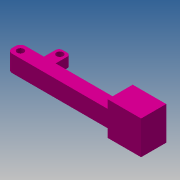
# Autodesk Inventor part: 連趕2
Saved by Autodesk Inventor 2015 (Build 190159000, 159)
## iProperties
Created: 2017-12-21
Part Number: 連趕2
Material: 一般
Document SubType Name: Modeling
Designer: user
Density: 1 g/cm^3
Appearance: 預設
Author: user
Autodesk Inventor part; units mm, degrees
ref_plane "YZ Plane" through (0, 0, 0) normal (1, 0, 0) x (0, 1, 0)
ref_plane "XZ Plane" through (0, 0, 0) normal (0, 1, 0) x (-1, 0, 0)
ref_plane "XY Plane" through (0, 0, 0) normal (0, 0, 1) x (1, 0, 0)
sketch "草圖1" plane through (0, 0, 0) normal (0, 0, 1) x (1, 0, 0)
  line L0 (0, 0) -> (80, 0)
  line L1 (80, 0) -> (80, 8)
  line L2 (60, 8) -> (0, 8)
  line L3 (0, 8) -> (0, 0)
  line L4 (80, 8) -> (60, 8)
  line L5 (60, 8) -> (60, 15)
  line L6 (60, 15) -> (80, 15)
  line L7 (80, 15) -> (80, 8)
  dimension "d0" = 80
  dimension "d1" = 20
  dimension "d2" = 15
  dimension "d3" = 8
  constraints: 16 end point, 4 parallel, 2 horizontal, 2 perpendicular
  measures "d0" distance of L0.start L0.end
  measures "d1" distance of L5.end L6.end
  measures "d2" distance between parallel lines of L0 L6
  measures "d3" distance between parallel lines of L0 L2
extrude "擠出1" add sketch "草圖1" along normal mid plane 20
sketch "草圖2" plane through (0, 0, 0) normal (0, 0, 1) x (1, 0, 0)
  line L0 (70, 31.4394) -> (70, 8.5)
  line L1 (60, 15) -> (80, 15) projected
  line L2 (80, 0) -> (80, 15) projected
  arc A0 (70, 8.5) -> (77.5, 16) centre (70, 16) ccw
  line L3 (70, 16) -> (77.5, 16)
  point P0 (0, 0)
  dimension "d14" = 7.5
  dimension "d15" = 1
  dimension "d16" = 10
  constraints: 6 end point, 2 point on circle, 1 centre point, 1 horizontal, 1 point on line, 1 vertical
  measures "d14" radius of A0
  measures "d15" distance between parallel lines of L1 L3
  measures "d16" distance between parallel lines of L2 L0
sketch "草圖3" plane through (0, 8, -10) normal (0, 1, 0) x (1, 0, 0)
  line L0 (60, 0) -> (60, -20) projected
  line L1 (0, 0) -> (60, 0)
  line L2 (60, 0) -> (60, -5)
  line L3 (60, -5) -> (0, -5)
  line L4 (0, -5) -> (0, 0)
  line L5 (0, -20) -> (60, -20)
  line L6 (60, -20) -> (60, -15)
  line L7 (60, -15) -> (0, -15)
  line L8 (0, -15) -> (0, -20)
  line L9 (60, -20) -> (0, -20) projected
  point P0 (0, -10)
  dimension "d10" = 5
  dimension "d11" = 5
  constraints: 16 end point, 4 parallel, 3 point on line, 2 horizontal, 2 perpendicular, 1 collinear
  measures "d10" distance between parallel lines of L7 L5
  measures "d11" distance between parallel lines of L1 L3
extrude "擠出2" cut sketch "草圖3" against normal blind 20
revolve "迴轉2" cut sketch "草圖2" angle 360 about axis through (70, 31.4394, 0) along (0, -1, 0)
sketch "草圖4" plane through (0, 8, 5) normal (0, 1, 0) x (1, 0, 0)
  line L0 (12, 8) -> (19, 8)
  line L1 (19, 8) -> (19, 2)
  line L2 (19, 2) -> (12, 2)
  line L3 (12, 2) -> (12, 8)
  point P0 (0, 5)
  dimension "d34" = 3
  dimension "d35" = 6
  dimension "d36" = 7
  dimension "d37" = 12
  constraints: 8 end point, 2 parallel, 1 horizontal, 1 perpendicular
  measures "d34" distance from line of point (0, 5) L0
  measures "d35" distance of L0.end L1.end
  measures "d36" distance between parallel lines of L3 L1
  measures "d37" distance from line of point (0, 5) L3
extrude "擠出3" add sketch "草圖4" along normal blind 11
sketch "草圖7" plane through (12, 8, 3) normal (0, 0, 1) x (1, 0, 0)
  circle A0 centre (3.5, 8) radius 2
  line L0 (7, 0) -> (0, 0) projected
  line L1 (7, 0) -> (7, 11) projected
  line L2 (0, 11) -> (7, 11) projected
  line L3 (0, 0) -> (0, 11) projected
  point P0 (-12, -8)
  dimension "d38" = 3.5
  dimension "d39" = 4
  dimension "d40" = 3
  constraints: 1 centre point
  measures "d38" distance from line of A0.centre L1
  measures "d39" diameter of A0
  measures "d40" distance from line of A0.centre L2
extrude "擠出6" cut sketch "草圖7" against normal blind 10 contours A0
fillet "圓角3" radius 2 2 edges at (12, 19, 0) (19, 19, 0)
fillet "圓角2" radius 3 2 edges at (0, 8, 0) (0, 0, 0)
sketch "草圖6" plane through (60, 0, 5) normal (0, 0, 1) x (1, 0, 0)
  arc A0 (-57, 8) -> (-60, 5) centre (-57, 5) ccw projected
  arc A1 (-60, 3) -> (-57, 0) centre (-57, 3) ccw projected
  circle A2 centre (-56, 4) radius 2
  line L0 (-57, 8) -> (0, 8) projected
  line L1 (-60, 3) -> (-60, 5) projected
  point P0 (-60, 0)
  dimension "d29" = 4
  dimension "d30" = 4
  dimension "d31" = 4
  constraints: 1 centre point
  measures "d29" distance from line of A2.centre L0
  measures "d30" distance from line of L1 A2.centre
  measures "d31" diameter of A2
extrude "擠出5" cut sketch "草圖6" against normal through all
sketch "草圖10" plane through (0, 0, -10) normal (0, 0, -1) x (-1, 0, 0)
  circle A0 centre (-70, 18) radius 7.5
  line L0 (-60, 15) -> (-80, 15) projected
  point P0 (0, 0)
  dimension "d52" = 15
  dimension "d53" = 3
  constraints: 1 centre point
  measures "d52" diameter of A0
  measures "d53" distance from line of L0 A0.centre
extrude "擠出9" cut sketch "草圖10" against normal blind 7
